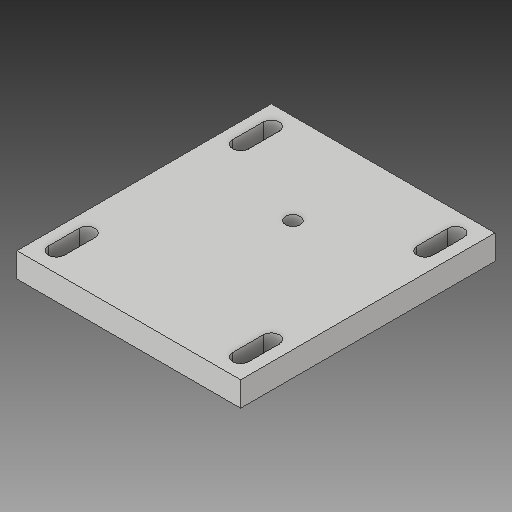
# Autodesk Inventor part: StepperAdapter
Saved by Autodesk Inventor 2019 (Build 230136000, 136)
## iProperties
Created: 2016-10-31
Part Number: StepperAdapter
Material: Generic
Document SubType Name: Modeling
Designer: Eivind
Density: 1 g/cm^3
Appearance: Default
Author: Eivind
Autodesk Inventor part; units mm, degrees
ref_plane "YZ Plane" through (0, 0, 0) normal (1, 0, 0) x (0, 1, 0)
ref_plane "XZ Plane" through (0, 0, 0) normal (0, 1, 0) x (-1, 0, 0)
ref_plane "XY Plane" through (0, 0, 0) normal (0, 0, 1) x (1, 0, 0)
sketch "Sketch2" plane through (0, 0, 0) normal (0, 1, 0) x (-1, 0, 0)
  arc A0 (21.75, 12.5) -> (28.25, 12.5) centre (25, 12.5) ccw
  line L0 (28.25, 12.5) -> (21.75, 12.5) construction
  line L1 (28.25, 12.5) -> (34.75, 12.5) construction
  line L2 (28.25, 12.5) -> (28.25, 25)
  line L3 (28.25, 12.5) -> (40.75, 12.5) construction
  line L4 (21.75, 12.5) -> (21.75, 25)
  line L5 (21.75, 12.5) -> (34.25, 12.5) construction
  arc A1 (28.25, 25) -> (21.75, 25) centre (25, 25) ccw
  arc A2 (-53.25, 12.5) -> (-46.75, 12.5) centre (-50, 12.5) ccw
  line L6 (-46.75, 12.5) -> (-53.25, 12.5) construction
  line L7 (-46.75, 12.5) -> (-40.25, 12.5) construction
  line L8 (-46.75, 12.5) -> (-46.75, 25)
  line L9 (-46.75, 12.5) -> (-34.25, 12.5) construction
  line L10 (-53.25, 12.5) -> (-53.25, 25)
  line L11 (-53.25, 12.5) -> (-40.75, 12.5) construction
  arc A3 (-46.75, 25) -> (-53.25, 25) centre (-50, 25) ccw
  arc A4 (-53.25, -62.5) -> (-46.75, -62.5) centre (-50, -62.5) ccw
  line L12 (-46.75, -62.5) -> (-53.25, -62.5) construction
  line L13 (-46.75, -62.5) -> (-40.25, -62.5) construction
  line L14 (-46.75, -62.5) -> (-46.75, -50)
  line L15 (-46.75, -62.5) -> (-34.25, -62.5) construction
  line L16 (-53.25, -62.5) -> (-53.25, -50)
  line L17 (-53.25, -62.5) -> (-40.75, -62.5) construction
  arc A5 (-46.75, -50) -> (-53.25, -50) centre (-50, -50) ccw
  line L18 (28.25, -62.5) -> (40.75, -62.5) construction
  line L19 (28.25, -62.5) -> (34.75, -62.5) construction
  line L20 (28.25, -62.5) -> (28.25, -50)
  line L21 (21.75, -62.5) -> (34.25, -62.5) construction
  arc A6 (21.75, -62.5) -> (28.25, -62.5) centre (25, -62.5) ccw
  line L22 (28.25, -62.5) -> (21.75, -62.5) construction
  line L23 (21.75, -62.5) -> (21.75, -50)
  arc A7 (28.25, -50) -> (21.75, -50) centre (25, -50) ccw
  line L24 (33, 33) -> (-58, 33)
  line L25 (-58, 33) -> (-58, -70.5)
  line L26 (-58, -70.5) -> (33, -70.5)
  line L27 (33, -70.5) -> (33, 33)
  circle A8 centre (-12.5, -33.75) radius 3
  point P0 (0, 0)
  dimension "d25" = 6.5
  dimension "d26" = 180
  dimension "d27" = 3.25
  dimension "d28" = 12.5
  dimension "d29" = 90
  dimension "d30" = 12.5
  dimension "d31" = 90
  dimension "d32" = 3.25
  dimension "d33" = 6.5
  dimension "d34" = 180
  dimension "d35" = 3.25
  dimension "d36" = 12.5
  dimension "d37" = 90
  dimension "d38" = 12.5
  dimension "d39" = 90
  dimension "d40" = 3.25
  dimension "d41" = 25
  dimension "d42" = 25
  dimension "d43" = 6.5
  dimension "d44" = 180
  dimension "d45" = 3.25
  dimension "d46" = 12.5
  dimension "d47" = 90
  dimension "d48" = 12.5
  dimension "d49" = 90
  dimension "d50" = 3.25
  dimension "d51" = 6.5
  dimension "d52" = 180
  dimension "d53" = 3.25
  dimension "d54" = 12.5
  dimension "d55" = 90
  dimension "d56" = 12.5
  dimension "d57" = 90
  dimension "d58" = 3.25
  dimension "d59" = 75
  dimension "d60" = 0
  dimension "d61" = 75
  dimension "d62" = 0
  dimension "d63" = 75
  dimension "d64" = 75
  dimension "d65" = 8
  dimension "d66" = 8
  dimension "d67" = 8
  dimension "d68" = 8
  dimension "d71" = 6
  dimension "d76" = 16.25
  dimension "d77" = 37.5
  constraints: 56 end point, 16 point on circle, 13 horizontal, 12 equal length, 9 centre point, 8 vertical, 2 parallel, 1 perpendicular
  measures "d25" distance of L0.start L0.end
  measures "d26" angle of L0 L1
  measures "d27" radius of A0
  measures "d28" distance of L0.start L2.end
  measures "d29" angle of L3 L2
  measures "d30" distance of L0.end L4.end
  measures "d31" angle of L5 L4
  measures "d32" radius of A1
  measures "d33" distance of L6.start L6.end
  measures "d34" angle of L6 L7
  measures "d35" radius of A2
  measures "d36" distance of L6.start L8.end
  measures "d37" angle of L9 L8
  measures "d38" distance of L6.end L10.end
  measures "d39" angle of L11 L10
  measures "d40" radius of A3
  measures "d41" horizontal distance of point (0, 0) A1.centre
  measures "d42" horizontal distance of point (0, 0) A1.centre
  measures "d43" distance of L15.start L17.start
  measures "d44" angle of L12 L13
  measures "d45" radius of A4
  measures "d46" distance of L15.start L14.end
  measures "d47" angle of L15 L14
  measures "d48" distance of L17.start L16.end
  measures "d49" angle of L17 L16
  measures "d50" radius of A5
  measures "d51" distance of L20.start L23.start
  measures "d52" angle of L22 L19
  measures "d53" radius of A6
  measures "d54" distance of L20.start L20.end
  measures "d55" angle of L18 L20
  measures "d56" distance of L23.start L23.end
  measures "d57" angle of L21 L23
  measures "d58" radius of A7
  measures "d59" distance of A3.centre A1.centre
  measures "d60" vertical distance of A3.centre A1.centre
  measures "d61" distance of A7.centre A1.centre
  measures "d62" horizontal distance of A1.centre A7.centre
  measures "d63" distance of A7.centre A5.centre
  measures "d64" distance of A5.centre A3.centre
  measures "d65" distance from line of L27 A1.centre
  measures "d66" distance from line of L24 A1.centre
  measures "d67" distance from line of L26 A6.centre
  measures "d68" distance from line of L25 A3.centre
  measures "d71" diameter of A8
  measures "d76" vertical distance of A5.centre A8.centre
  measures "d77" horizontal distance of A7.centre A8.centre
extrude "Extrusion2" add sketch "Sketch2" along normal blind 10
body "Solid2"
